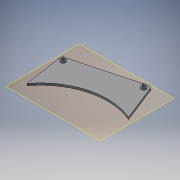
# Autodesk Inventor part: housing_undercover
Saved by Autodesk Inventor 2017 (Build 210142000, 142)
## iProperties
Created: 2017-06-11
Part Number: housing_undercover
Material: Ogólny
Document SubType Name: Modeling
Designer: Speed King
Density: 1 g/cm^3
Appearance: Domyślna
Author: Speed King
Autodesk Inventor part; units mm, degrees
ref_plane "YZ Plane" through (0, 0, 0) normal (1, 0, 0) x (0, 1, 0)
ref_plane "XZ Plane" through (0, 0, 0) normal (0, 1, 0) x (-1, 0, 0)
ref_plane "XY Plane" through (0, 0, 0) normal (0, 0, 1) x (1, 0, 0)
ref_plane "Płaszczyzna konstrukcyjna1" through (0, 0, 0) normal (0, 0, 1) x (1, 0, 0)
sketch "Szkic1" plane through (0, 0, 0) normal (0, 0, 1) x (1, 0, 0)
  line L0 (-77.9596, -24.5647) -> (-89.3248, 51.2994) projected
  arc A0 (-85.674, 56.8699) -> (-89.3248, 51.2994) centre (-84.3799, 52.0402) ccw projected
  line L1 (-85.674, 56.8699) -> (45.761, 92.0878) projected
  arc A1 (51.7078, 89.089) -> (45.761, 92.0878) centre (47.0551, 87.2581) ccw projected
  line L2 (51.7078, 89.089) -> (79.7973, 17.7061) projected
  circle A2 centre (27.7277, -103.4811) radius 131.9 projected
  line L3 (-77.9596, -24.5647) -> (-89.3248, 51.2994)
  line L4 (79.7973, 17.7061) -> (51.7078, 89.089)
  arc A3 (79.7973, 17.7061) -> (-77.9596, -24.5647) centre (27.7277, -103.4811) ccw
  arc A4 (-85.674, 56.8699) -> (-89.3248, 51.2994) centre (-84.3799, 52.0402) ccw
  arc A5 (51.7078, 89.089) -> (45.761, 92.0878) centre (47.0551, 87.2581) ccw
  line L5 (-85.674, 56.8699) -> (45.761, 92.0878)
  point P0 (0, 0)
  constraints: 6 end point, 6 point on circle, 4 tangent, 3 centre point, 2 collinear, 1 point on line, 3 other
extrude "Wyciągnięcie proste1" add sketch "Szkic1" along normal blind 4 contours L0 A0 L1 A1 L2 A2
sketch "Szkic2" plane through (0, 0, 4) normal (0, 0, 1) x (1, 0, 0)
  circle A0 centre (-80.4123, 48.9622) radius 5
  line L0 (-37.9291, 141.5533) -> (24.1284, -90.0484) construction
  line L1 (45.761, 92.0878) -> (-85.674, 56.8699) construction
  circle A1 centre (45.158, 82.6087) radius 5
  point P0 (0, 0)
  dimension "d2" = 10
  dimension "d3" = 65
  dimension "d4" = 9
  constraints: 2 centre point, 2 end point, 1 symmetric about line, 4 other
  measures "d2" diameter of A0
  measures "d3" distance from line of L0 A0.centre
  measures "d4" distance from line of A0.centre L1
extrude "Wyciągnięcie proste2" add sketch "Szkic2" along normal blind 4
sketch "Szkic3" plane through (45.158, 82.6087, 8) normal (0, 0, 1) x (1, 0, 0)
  circle A0 centre (0, 0) radius 5 projected
  circle A1 centre (-125.5704, -33.6465) radius 5 projected
  line L0 (-124.7784, -30.6908) -> (-122.6147, -32.8545)
  line L1 (-122.6147, -32.8545) -> (-123.4066, -35.8102)
  line L2 (-123.4066, -35.8102) -> (-126.3623, -36.6022)
  line L3 (-126.3623, -36.6022) -> (-128.526, -34.4385)
  line L4 (-128.526, -34.4385) -> (-127.7341, -31.4828)
  line L5 (-127.7341, -31.4828) -> (-124.7784, -30.6908)
  line L6 (0.792, 2.9557) -> (2.9557, 0.792)
  line L7 (2.9557, 0.792) -> (2.1637, -2.1637)
  line L8 (2.1637, -2.1637) -> (-0.792, -2.9557)
  line L9 (-0.792, -2.9557) -> (-2.9557, -0.792)
  line L10 (-2.9557, -0.792) -> (-2.1637, 2.1637)
  line L11 (-2.1637, 2.1637) -> (0.792, 2.9557)
  line L12 (0.6029, 9.479) -> (-130.832, -25.7389) projected
  point P0 (-45.158, -82.6087)
  dimension "d7" = 5.3
  dimension "d8" = 5.3
  constraints: 24 end point, 2 coincident, 2 parallel, 26 other
  measures "d7" distance between parallel lines of L8 L11
  measures "d8" distance between parallel lines of L2 L5
extrude "Wyciągnięcie proste3" cut sketch "Szkic3" against normal blind 2.5 contours L0 L1 L2 L3 L4 L5 | L6 L7 L8 L9 L10 L11
sketch "Szkic4" plane through (45.158, 82.6087, 5.5) normal (0, 0, 1) x (1, 0, 0)
  circle A0 centre (0, 0) radius 5 projected
  circle A1 centre (-125.5704, -33.6465) radius 5 projected
  circle A2 centre (0, 0) radius 1.35
  circle A3 centre (-125.5704, -33.6465) radius 1.35
  point P0 (-45.158, -82.6087)
  dimension "d11" = 2.7
  dimension "d12" = 2.7
  constraints: 2 centre point, 2 coincident
  measures "d11" diameter of A2
  measures "d12" diameter of A3
extrude "Wyciągnięcie proste4" cut sketch "Szkic4" against normal up to next contours A2 | A3
equation "\"d8\" = d7"
equation "\"d12\" = d11"
